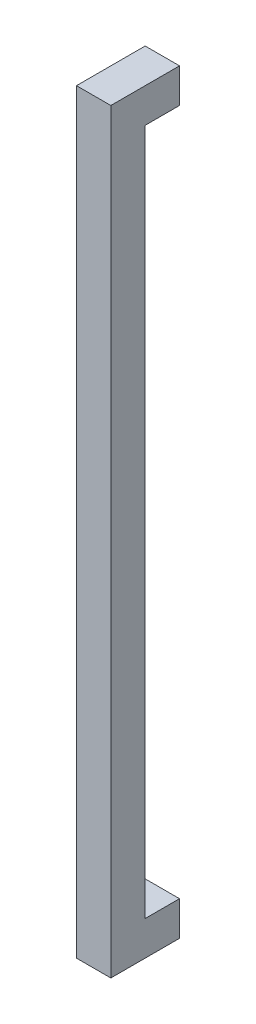
# Autodesk Inventor part: ReinforcerLarge
Saved by Autodesk Inventor 2027 (Build 310192000, 192)
## iProperties
Created: 2026-04-15
Part Number: ReinforcerLarge
Material: Generic
Document SubType Name: Modeling
Designer: Tueha
Density: 1 g/cm^3
Appearance: Default
Author: Tueha
Autodesk Inventor part; units mm, degrees
ref_plane "YZ Plane" through (0, 0, 0) normal (1, 0, 0) x (0, 1, 0)
ref_plane "XZ Plane" through (0, 0, 0) normal (0, 1, 0) x (-1, 0, 0)
ref_plane "XY Plane" through (0, 0, 0) normal (0, 0, 1) x (1, 0, 0)
sketch "Sketch1" plane through (0, 0, 0) normal (0, 0, 1) x (1, 0, 0)
  line L0 (538.5222, 35.1205) -> (532.3222, 35.1205) projected
  line L1 (538.5222, 52.0205) -> (538.5222, 35.1205) projected
  line L2 (538.5222, 52.0205) -> (246.9222, 52.0205) projected
  line L3 (246.9222, 52.0205) -> (246.9222, 58.0205) projected
  line L4 (246.9222, 58.0205) -> (538.5222, 58.0205) projected
  line L5 (538.5222, 74.9205) -> (538.5222, 58.0205) projected
  line L6 (523.1184, 74.9205) -> (538.5222, 74.9205) projected
  line L7 (517.9222, 77.9205) -> (523.1184, 74.9205) projected
  line L8 (517.9222, 74.9205) -> (517.9222, 77.9205) projected
  arc A0 (515.9222, 74.9205) -> (517.9222, 74.9205) centre (516.9222, 74.9205) ccw projected
  line L9 (515.9222, 77.9205) -> (515.9222, 74.9205) projected
  line L10 (510.7261, 74.9205) -> (515.9222, 77.9205) projected
  line L11 (494.3184, 74.9205) -> (510.7261, 74.9205) projected
  line L12 (489.1222, 77.9205) -> (494.3184, 74.9205) projected
  line L13 (489.1222, 74.9205) -> (489.1222, 77.9205) projected
  arc A1 (487.1222, 74.9205) -> (489.1222, 74.9205) centre (488.1222, 74.9205) ccw projected
  line L14 (487.1222, 77.9205) -> (487.1222, 74.9205) projected
  line L15 (481.9261, 74.9205) -> (487.1222, 77.9205) projected
  line L16 (465.5184, 74.9205) -> (481.9261, 74.9205) projected
  line L17 (460.3222, 77.9205) -> (465.5184, 74.9205) projected
  line L18 (460.3222, 74.9205) -> (460.3222, 77.9205) projected
  arc A2 (458.3222, 74.9205) -> (460.3222, 74.9205) centre (459.3222, 74.9205) ccw projected
  line L19 (458.3222, 77.9205) -> (458.3222, 74.9205) projected
  line L20 (453.1261, 74.9205) -> (458.3222, 77.9205) projected
  line L21 (436.7184, 74.9205) -> (453.1261, 74.9205) projected
  line L22 (431.5222, 77.9205) -> (436.7184, 74.9205) projected
  line L23 (431.5222, 74.9205) -> (431.5222, 77.9205) projected
  arc A3 (429.5222, 74.9205) -> (431.5222, 74.9205) centre (430.5222, 74.9205) ccw projected
  line L24 (429.5222, 77.9205) -> (429.5222, 74.9205) projected
  line L25 (424.3261, 74.9205) -> (429.5222, 77.9205) projected
  line L26 (407.9184, 74.9205) -> (424.3261, 74.9205) projected
  line L27 (402.7222, 77.9205) -> (407.9184, 74.9205) projected
  line L28 (402.7222, 74.9205) -> (402.7222, 77.9205) projected
  arc A4 (400.7222, 74.9205) -> (402.7222, 74.9205) centre (401.7222, 74.9205) ccw projected
  line L29 (400.7222, 77.9205) -> (400.7222, 74.9205) projected
  line L30 (395.5261, 74.9205) -> (400.7222, 77.9205) projected
  line L31 (379.1184, 74.9205) -> (395.5261, 74.9205) projected
  line L32 (373.9222, 77.9205) -> (379.1184, 74.9205) projected
  line L33 (373.9222, 74.9205) -> (373.9222, 77.9205) projected
  arc A5 (371.9222, 74.9205) -> (373.9222, 74.9205) centre (372.9222, 74.9205) ccw projected
  line L34 (371.9222, 77.9205) -> (371.9222, 74.9205) projected
  line L35 (366.7261, 74.9205) -> (371.9222, 77.9205) projected
  line L36 (350.3184, 74.9205) -> (366.7261, 74.9205) projected
  line L37 (345.1222, 77.9205) -> (350.3184, 74.9205) projected
  line L38 (345.1222, 74.9205) -> (345.1222, 77.9205) projected
  arc A6 (343.1222, 74.9205) -> (345.1222, 74.9205) centre (344.1222, 74.9205) ccw projected
  line L39 (343.1222, 77.9205) -> (343.1222, 74.9205) projected
  line L40 (337.9261, 74.9205) -> (343.1222, 77.9205) projected
  line L41 (321.5184, 74.9205) -> (337.9261, 74.9205) projected
  line L42 (316.3222, 77.9205) -> (321.5184, 74.9205) projected
  line L43 (316.3222, 74.9205) -> (316.3222, 77.9205) projected
  arc A7 (314.3222, 74.9205) -> (316.3222, 74.9205) centre (315.3222, 74.9205) ccw projected
  line L44 (314.3222, 77.9205) -> (314.3222, 74.9205) projected
  line L45 (309.1261, 74.9205) -> (314.3222, 77.9205) projected
  line L46 (292.7184, 74.9205) -> (309.1261, 74.9205) projected
  line L47 (287.5222, 77.9205) -> (292.7184, 74.9205) projected
  line L48 (287.5222, 74.9205) -> (287.5222, 77.9205) projected
  arc A8 (285.5222, 74.9205) -> (287.5222, 74.9205) centre (286.5222, 74.9205) ccw projected
  line L49 (285.5222, 77.9205) -> (285.5222, 74.9205) projected
  line L50 (280.3261, 74.9205) -> (285.5222, 77.9205) projected
  line L51 (263.9184, 74.9205) -> (280.3261, 74.9205) projected
  line L52 (258.7222, 77.9205) -> (263.9184, 74.9205) projected
  line L53 (258.7222, 74.9205) -> (258.7222, 77.9205) projected
  arc A9 (256.7222, 74.9205) -> (258.7222, 74.9205) centre (257.7222, 74.9205) ccw projected
  line L54 (256.7222, 77.9205) -> (256.7222, 74.9205) projected
  line L55 (251.5261, 74.9205) -> (256.7222, 77.9205) projected
  line L56 (235.1184, 74.9205) -> (251.5261, 74.9205) projected
  line L57 (229.9222, 77.9205) -> (235.1184, 74.9205) projected
  line L58 (229.9222, 74.9205) -> (229.9222, 77.9205) projected
  arc A10 (227.9222, 74.9205) -> (229.9222, 74.9205) centre (228.9222, 74.9205) ccw projected
  line L59 (227.9222, 77.9205) -> (227.9222, 74.9205) projected
  line L60 (222.7261, 74.9205) -> (227.9222, 77.9205) projected
  line L61 (206.3184, 74.9205) -> (222.7261, 74.9205) projected
  line L62 (201.1222, 77.9205) -> (206.3184, 74.9205) projected
  line L63 (201.1222, 74.9205) -> (201.1222, 77.9205) projected
  arc A11 (199.1222, 74.9205) -> (201.1222, 74.9205) centre (200.1222, 74.9205) ccw projected
  line L64 (199.1222, 77.9205) -> (199.1222, 74.9205) projected
  line L65 (193.9261, 74.9205) -> (199.1222, 77.9205) projected
  line L66 (177.5184, 74.9205) -> (193.9261, 74.9205) projected
  line L67 (172.3222, 77.9205) -> (177.5184, 74.9205) projected
  line L68 (172.3222, 74.9205) -> (172.3222, 77.9205) projected
  arc A12 (170.3222, 74.9205) -> (172.3222, 74.9205) centre (171.3222, 74.9205) ccw projected
  line L69 (170.3222, 77.9205) -> (170.3222, 74.9205) projected
  line L70 (165.1261, 74.9205) -> (170.3222, 77.9205) projected
  line L71 (148.7184, 74.9205) -> (165.1261, 74.9205) projected
  line L72 (143.5222, 77.9205) -> (148.7184, 74.9205) projected
  line L73 (143.5222, 74.9205) -> (143.5222, 77.9205) projected
  arc A13 (141.5222, 74.9205) -> (143.5222, 74.9205) centre (142.5222, 74.9205) ccw projected
  line L74 (141.5222, 77.9205) -> (141.5222, 74.9205) projected
  line L75 (136.3261, 74.9205) -> (141.5222, 77.9205) projected
  line L76 (119.9184, 74.9205) -> (136.3261, 74.9205) projected
  line L77 (114.7222, 77.9205) -> (119.9184, 74.9205) projected
  line L78 (114.7222, 74.9205) -> (114.7222, 77.9205) projected
  arc A14 (112.7222, 74.9205) -> (114.7222, 74.9205) centre (113.7222, 74.9205) ccw projected
  line L79 (112.7222, 77.9205) -> (112.7222, 74.9205) projected
  line L80 (107.5261, 74.9205) -> (112.7222, 77.9205) projected
  line L81 (91.1184, 74.9205) -> (107.5261, 74.9205) projected
  line L82 (85.9222, 77.9205) -> (91.1184, 74.9205) projected
  line L83 (85.9222, 74.9205) -> (85.9222, 77.9205) projected
  arc A15 (83.9222, 74.9205) -> (85.9222, 74.9205) centre (84.9222, 74.9205) ccw projected
  line L84 (83.9222, 77.9205) -> (83.9222, 74.9205) projected
  line L85 (78.7261, 74.9205) -> (83.9222, 77.9205) projected
  line L86 (62.3184, 74.9205) -> (78.7261, 74.9205) projected
  line L87 (57.1222, 77.9205) -> (62.3184, 74.9205) projected
  line L88 (57.1222, 74.9205) -> (57.1222, 77.9205) projected
  arc A16 (55.1222, 74.9205) -> (57.1222, 74.9205) centre (56.1222, 74.9205) ccw projected
  line L89 (55.1222, 77.9205) -> (55.1222, 74.9205) projected
  line L90 (49.9261, 74.9205) -> (55.1222, 77.9205) projected
  line L91 (33.5184, 74.9205) -> (49.9261, 74.9205) projected
  line L92 (28.3222, 77.9205) -> (33.5184, 74.9205) projected
  line L93 (28.3222, 74.9205) -> (28.3222, 77.9205) projected
  arc A17 (26.3222, 74.9205) -> (28.3222, 74.9205) centre (27.3222, 74.9205) ccw projected
  line L94 (26.3222, 77.9205) -> (26.3222, 74.9205) projected
  line L95 (21.1261, 74.9205) -> (26.3222, 77.9205) projected
  line L96 (4.7184, 74.9205) -> (21.1261, 74.9205) projected
  line L97 (-0.4778, 77.9205) -> (4.7184, 74.9205) projected
  line L98 (-0.4778, 74.9205) -> (-0.4778, 77.9205) projected
  arc A18 (-2.4778, 74.9205) -> (-0.4778, 74.9205) centre (-1.4778, 74.9205) ccw projected
  line L99 (-2.4778, 77.9205) -> (-2.4778, 74.9205) projected
  line L100 (-7.6739, 74.9205) -> (-2.4778, 77.9205) projected
  line L101 (-24.0816, 74.9205) -> (-7.6739, 74.9205) projected
  line L102 (-29.2778, 77.9205) -> (-24.0816, 74.9205) projected
  line L103 (-29.2778, 74.9205) -> (-29.2778, 77.9205) projected
  arc A19 (-31.2778, 74.9205) -> (-29.2778, 74.9205) centre (-30.2778, 74.9205) ccw projected
  line L104 (-31.2778, 77.9205) -> (-31.2778, 74.9205) projected
  line L105 (-36.4739, 74.9205) -> (-31.2778, 77.9205) projected
  line L106 (-36.4739, 74.9205) -> (-44.6778, 74.9205) projected
  line L107 (-44.6778, 35.1205) -> (-44.6778, 74.9205) projected
  line L108 (-22.0739, 35.1205) -> (-44.6778, 35.1205) projected
  line L109 (-16.8778, 32.1205) -> (-22.0739, 35.1205) projected
  line L110 (-16.8778, 35.1205) -> (-16.8778, 32.1205) projected
  arc A20 (-14.8778, 35.1205) -> (-16.8778, 35.1205) centre (-15.8778, 35.1205) ccw projected
  line L111 (-14.8778, 32.1205) -> (-14.8778, 35.1205) projected
  line L112 (-9.6816, 35.1205) -> (-14.8778, 32.1205) projected
  line L113 (6.7261, 35.1205) -> (-9.6816, 35.1205) projected
  line L114 (11.9222, 32.1205) -> (6.7261, 35.1205) projected
  line L115 (11.9222, 35.1205) -> (11.9222, 32.1205) projected
  arc A21 (13.9222, 35.1205) -> (11.9222, 35.1205) centre (12.9222, 35.1205) ccw projected
  line L116 (13.9222, 32.1205) -> (13.9222, 35.1205) projected
  line L117 (19.1184, 35.1205) -> (13.9222, 32.1205) projected
  line L118 (35.5261, 35.1205) -> (19.1184, 35.1205) projected
  line L119 (40.7222, 32.1205) -> (35.5261, 35.1205) projected
  line L120 (40.7222, 35.1205) -> (40.7222, 32.1205) projected
  arc A22 (42.7222, 35.1205) -> (40.7222, 35.1205) centre (41.7222, 35.1205) ccw projected
  line L121 (42.7222, 32.1205) -> (42.7222, 35.1205) projected
  line L122 (47.9184, 35.1205) -> (42.7222, 32.1205) projected
  line L123 (64.3261, 35.1205) -> (47.9184, 35.1205) projected
  line L124 (69.5222, 32.1205) -> (64.3261, 35.1205) projected
  line L125 (69.5222, 35.1205) -> (69.5222, 32.1205) projected
  arc A23 (71.5222, 35.1205) -> (69.5222, 35.1205) centre (70.5222, 35.1205) ccw projected
  line L126 (71.5222, 32.1205) -> (71.5222, 35.1205) projected
  line L127 (76.7184, 35.1205) -> (71.5222, 32.1205) projected
  line L128 (93.1261, 35.1205) -> (76.7184, 35.1205) projected
  line L129 (98.3222, 32.1205) -> (93.1261, 35.1205) projected
  line L130 (98.3222, 35.1205) -> (98.3222, 32.1205) projected
  arc A24 (100.3222, 35.1205) -> (98.3222, 35.1205) centre (99.3222, 35.1205) ccw projected
  line L131 (100.3222, 32.1205) -> (100.3222, 35.1205) projected
  line L132 (105.5184, 35.1205) -> (100.3222, 32.1205) projected
  line L133 (121.9261, 35.1205) -> (105.5184, 35.1205) projected
  line L134 (127.1222, 32.1205) -> (121.9261, 35.1205) projected
  line L135 (127.1222, 35.1205) -> (127.1222, 32.1205) projected
  arc A25 (129.1222, 35.1205) -> (127.1222, 35.1205) centre (128.1222, 35.1205) ccw projected
  line L136 (129.1222, 32.1205) -> (129.1222, 35.1205) projected
  line L137 (134.3184, 35.1205) -> (129.1222, 32.1205) projected
  line L138 (150.7261, 35.1205) -> (134.3184, 35.1205) projected
  line L139 (155.9222, 32.1205) -> (150.7261, 35.1205) projected
  line L140 (155.9222, 35.1205) -> (155.9222, 32.1205) projected
  arc A26 (157.9222, 35.1205) -> (155.9222, 35.1205) centre (156.9222, 35.1205) ccw projected
  line L141 (157.9222, 32.1205) -> (157.9222, 35.1205) projected
  line L142 (163.1184, 35.1205) -> (157.9222, 32.1205) projected
  line L143 (179.5261, 35.1205) -> (163.1184, 35.1205) projected
  line L144 (184.7222, 32.1205) -> (179.5261, 35.1205) projected
  line L145 (184.7222, 35.1205) -> (184.7222, 32.1205) projected
  arc A27 (186.7222, 35.1205) -> (184.7222, 35.1205) centre (185.7222, 35.1205) ccw projected
  line L146 (186.7222, 32.1205) -> (186.7222, 35.1205) projected
  line L147 (191.9184, 35.1205) -> (186.7222, 32.1205) projected
  line L148 (208.3261, 35.1205) -> (191.9184, 35.1205) projected
  line L149 (213.5222, 32.1205) -> (208.3261, 35.1205) projected
  line L150 (213.5222, 35.1205) -> (213.5222, 32.1205) projected
  arc A28 (215.5222, 35.1205) -> (213.5222, 35.1205) centre (214.5222, 35.1205) ccw projected
  line L151 (215.5222, 32.1205) -> (215.5222, 35.1205) projected
  line L152 (220.7184, 35.1205) -> (215.5222, 32.1205) projected
  line L153 (237.1261, 35.1205) -> (220.7184, 35.1205) projected
  line L154 (242.3222, 32.1205) -> (237.1261, 35.1205) projected
  line L155 (242.3222, 35.1205) -> (242.3222, 32.1205) projected
  arc A29 (244.3222, 35.1205) -> (242.3222, 35.1205) centre (243.3222, 35.1205) ccw projected
  line L156 (244.3222, 32.1205) -> (244.3222, 35.1205) projected
  line L157 (249.5184, 35.1205) -> (244.3222, 32.1205) projected
  line L158 (265.9261, 35.1205) -> (249.5184, 35.1205) projected
  line L159 (271.1222, 32.1205) -> (265.9261, 35.1205) projected
  line L160 (271.1222, 35.1205) -> (271.1222, 32.1205) projected
  arc A30 (273.1222, 35.1205) -> (271.1222, 35.1205) centre (272.1222, 35.1205) ccw projected
  line L161 (273.1222, 32.1205) -> (273.1222, 35.1205) projected
  line L162 (278.3184, 35.1205) -> (273.1222, 32.1205) projected
  line L163 (294.7261, 35.1205) -> (278.3184, 35.1205) projected
  line L164 (299.9222, 32.1205) -> (294.7261, 35.1205) projected
  line L165 (299.9222, 35.1205) -> (299.9222, 32.1205) projected
  arc A31 (301.9222, 35.1205) -> (299.9222, 35.1205) centre (300.9222, 35.1205) ccw projected
  line L166 (301.9222, 32.1205) -> (301.9222, 35.1205) projected
  line L167 (307.1184, 35.1205) -> (301.9222, 32.1205) projected
  line L168 (323.5261, 35.1205) -> (307.1184, 35.1205) projected
  line L169 (328.7222, 32.1205) -> (323.5261, 35.1205) projected
  line L170 (328.7222, 35.1205) -> (328.7222, 32.1205) projected
  arc A32 (330.7222, 35.1205) -> (328.7222, 35.1205) centre (329.7222, 35.1205) ccw projected
  line L171 (330.7222, 32.1205) -> (330.7222, 35.1205) projected
  line L172 (335.9184, 35.1205) -> (330.7222, 32.1205) projected
  line L173 (352.3261, 35.1205) -> (335.9184, 35.1205) projected
  line L174 (357.5222, 32.1205) -> (352.3261, 35.1205) projected
  line L175 (357.5222, 35.1205) -> (357.5222, 32.1205) projected
  arc A33 (359.5222, 35.1205) -> (357.5222, 35.1205) centre (358.5222, 35.1205) ccw projected
  line L176 (359.5222, 32.1205) -> (359.5222, 35.1205) projected
  line L177 (364.7184, 35.1205) -> (359.5222, 32.1205) projected
  line L178 (381.1261, 35.1205) -> (364.7184, 35.1205) projected
  line L179 (386.3222, 32.1205) -> (381.1261, 35.1205) projected
  line L180 (386.3222, 35.1205) -> (386.3222, 32.1205) projected
  arc A34 (388.3222, 35.1205) -> (386.3222, 35.1205) centre (387.3222, 35.1205) ccw projected
  line L181 (388.3222, 32.1205) -> (388.3222, 35.1205) projected
  line L182 (393.5184, 35.1205) -> (388.3222, 32.1205) projected
  line L183 (409.9261, 35.1205) -> (393.5184, 35.1205) projected
  line L184 (415.1222, 32.1205) -> (409.9261, 35.1205) projected
  line L185 (415.1222, 35.1205) -> (415.1222, 32.1205) projected
  arc A35 (417.1222, 35.1205) -> (415.1222, 35.1205) centre (416.1222, 35.1205) ccw projected
  line L186 (417.1222, 32.1205) -> (417.1222, 35.1205) projected
  line L187 (422.3184, 35.1205) -> (417.1222, 32.1205) projected
  line L188 (438.7261, 35.1205) -> (422.3184, 35.1205) projected
  line L189 (443.9222, 32.1205) -> (438.7261, 35.1205) projected
  line L190 (443.9222, 35.1205) -> (443.9222, 32.1205) projected
  arc A36 (445.9222, 35.1205) -> (443.9222, 35.1205) centre (444.9222, 35.1205) ccw projected
  line L191 (445.9222, 32.1205) -> (445.9222, 35.1205) projected
  line L192 (451.1184, 35.1205) -> (445.9222, 32.1205) projected
  line L193 (467.5261, 35.1205) -> (451.1184, 35.1205) projected
  line L194 (472.7222, 32.1205) -> (467.5261, 35.1205) projected
  line L195 (472.7222, 35.1205) -> (472.7222, 32.1205) projected
  arc A37 (474.7222, 35.1205) -> (472.7222, 35.1205) centre (473.7222, 35.1205) ccw projected
  line L196 (474.7222, 32.1205) -> (474.7222, 35.1205) projected
  line L197 (479.9184, 35.1205) -> (474.7222, 32.1205) projected
  line L198 (496.3261, 35.1205) -> (479.9184, 35.1205) projected
  line L199 (501.5222, 32.1205) -> (496.3261, 35.1205) projected
  line L200 (501.5222, 35.1205) -> (501.5222, 32.1205) projected
  arc A38 (503.5222, 35.1205) -> (501.5222, 35.1205) centre (502.5222, 35.1205) ccw projected
  line L201 (503.5222, 32.1205) -> (503.5222, 35.1205) projected
  line L202 (508.7184, 35.1205) -> (503.5222, 32.1205) projected
  line L203 (525.1261, 35.1205) -> (508.7184, 35.1205) projected
  line L204 (530.3222, 32.1205) -> (525.1261, 35.1205) projected
  line L205 (530.3222, 35.1205) -> (530.3222, 32.1205) projected
  arc A39 (532.3222, 35.1205) -> (530.3222, 35.1205) centre (531.3222, 35.1205) ccw projected
  line L206 (-15.2778, 46.0205) -> (-9.2778, 46.0205) projected
  line L207 (-9.2778, 46.0205) -> (-9.2778, 40.0205) projected
  line L208 (-9.2778, 40.0205) -> (-15.2778, 40.0205) projected
  line L209 (-15.2778, 40.0205) -> (-15.2778, 46.0205) projected
  line L210 (-15.2778, 64.0205) -> (-15.2778, 70.0205) projected
  line L211 (-15.2778, 70.0205) -> (-9.2778, 70.0205) projected
  line L212 (-9.2778, 70.0205) -> (-9.2778, 64.0205) projected
  line L213 (-9.2778, 64.0205) -> (-15.2778, 64.0205) projected
  line L214 (42.3222, 46.0205) -> (48.3222, 46.0205) projected
  line L215 (48.3222, 46.0205) -> (48.3222, 40.0205) projected
  line L216 (48.3222, 40.0205) -> (42.3222, 40.0205) projected
  line L217 (42.3222, 40.0205) -> (42.3222, 46.0205) projected
  line L218 (42.3222, 64.0205) -> (42.3222, 70.0205) projected
  line L219 (42.3222, 70.0205) -> (48.3222, 70.0205) projected
  line L220 (48.3222, 70.0205) -> (48.3222, 64.0205) projected
  line L221 (48.3222, 64.0205) -> (42.3222, 64.0205) projected
  line L222 (99.9222, 46.0205) -> (105.9222, 46.0205) projected
  line L223 (105.9222, 46.0205) -> (105.9222, 40.0205) projected
  line L224 (105.9222, 40.0205) -> (99.9222, 40.0205) projected
  line L225 (99.9222, 40.0205) -> (99.9222, 46.0205) projected
  line L226 (99.9222, 64.0205) -> (99.9222, 70.0205) projected
  line L227 (99.9222, 70.0205) -> (105.9222, 70.0205) projected
  line L228 (105.9222, 70.0205) -> (105.9222, 64.0205) projected
  line L229 (105.9222, 64.0205) -> (99.9222, 64.0205) projected
  line L230 (157.5222, 46.0205) -> (163.5222, 46.0205) projected
  line L231 (163.5222, 46.0205) -> (163.5222, 40.0205) projected
  line L232 (163.5222, 40.0205) -> (157.5222, 40.0205) projected
  line L233 (157.5222, 40.0205) -> (157.5222, 46.0205) projected
  line L234 (157.5222, 64.0205) -> (157.5222, 70.0205) projected
  line L235 (157.5222, 70.0205) -> (163.5222, 70.0205) projected
  line L236 (163.5222, 70.0205) -> (163.5222, 64.0205) projected
  line L237 (163.5222, 64.0205) -> (157.5222, 64.0205) projected
  line L238 (215.1222, 46.0205) -> (221.1222, 46.0205) projected
  line L239 (221.1222, 46.0205) -> (221.1222, 40.0205) projected
  line L240 (221.1222, 40.0205) -> (215.1222, 40.0205) projected
  line L241 (215.1222, 40.0205) -> (215.1222, 46.0205) projected
  line L242 (215.1222, 64.0205) -> (215.1222, 70.0205) projected
  line L243 (215.1222, 70.0205) -> (221.1222, 70.0205) projected
  line L244 (221.1222, 70.0205) -> (221.1222, 64.0205) projected
  line L245 (221.1222, 64.0205) -> (215.1222, 64.0205) projected
  line L246 (272.7222, 46.0205) -> (278.7222, 46.0205) projected
  line L247 (278.7222, 46.0205) -> (278.7222, 40.0205) projected
  line L248 (278.7222, 40.0205) -> (272.7222, 40.0205) projected
  line L249 (272.7222, 40.0205) -> (272.7222, 46.0205) projected
  line L250 (272.7222, 64.0205) -> (272.7222, 70.0205) projected
  line L251 (272.7222, 70.0205) -> (278.7222, 70.0205) projected
  line L252 (278.7222, 70.0205) -> (278.7222, 64.0205) projected
  line L253 (278.7222, 64.0205) -> (272.7222, 64.0205) projected
  line L254 (330.3222, 46.0205) -> (336.3222, 46.0205) projected
  line L255 (336.3222, 46.0205) -> (336.3222, 40.0205) projected
  line L256 (336.3222, 40.0205) -> (330.3222, 40.0205) projected
  line L257 (330.3222, 40.0205) -> (330.3222, 46.0205) projected
  line L258 (330.3222, 64.0205) -> (330.3222, 70.0205) projected
  line L259 (330.3222, 70.0205) -> (336.3222, 70.0205) projected
  line L260 (336.3222, 70.0205) -> (336.3222, 64.0205) projected
  line L261 (336.3222, 64.0205) -> (330.3222, 64.0205) projected
  line L262 (387.9222, 46.0205) -> (393.9222, 46.0205) projected
  line L263 (393.9222, 46.0205) -> (393.9222, 40.0205) projected
  line L264 (393.9222, 40.0205) -> (387.9222, 40.0205) projected
  line L265 (387.9222, 40.0205) -> (387.9222, 46.0205) projected
  line L266 (387.9222, 64.0205) -> (387.9222, 70.0205) projected
  line L267 (387.9222, 70.0205) -> (393.9222, 70.0205) projected
  line L268 (393.9222, 70.0205) -> (393.9222, 64.0205) projected
  line L269 (393.9222, 64.0205) -> (387.9222, 64.0205) projected
  line L270 (445.5222, 46.0205) -> (451.5222, 46.0205) projected
  line L271 (451.5222, 46.0205) -> (451.5222, 40.0205) projected
  line L272 (451.5222, 40.0205) -> (445.5222, 40.0205) projected
  line L273 (445.5222, 40.0205) -> (445.5222, 46.0205) projected
  line L274 (445.5222, 64.0205) -> (445.5222, 70.0205) projected
  line L275 (445.5222, 70.0205) -> (451.5222, 70.0205) projected
  line L276 (451.5222, 70.0205) -> (451.5222, 64.0205) projected
  line L277 (451.5222, 64.0205) -> (445.5222, 64.0205) projected
  line L278 (503.1222, 46.0205) -> (509.1222, 46.0205) projected
  line L279 (509.1222, 46.0205) -> (509.1222, 40.0205) projected
  line L280 (509.1222, 40.0205) -> (503.1222, 40.0205) projected
  line L281 (503.1222, 40.0205) -> (503.1222, 46.0205) projected
  line L282 (503.1222, 64.0205) -> (503.1222, 70.0205) projected
  line L283 (503.1222, 70.0205) -> (509.1222, 70.0205) projected
  line L284 (509.1222, 70.0205) -> (509.1222, 64.0205) projected
  line L285 (509.1222, 64.0205) -> (503.1222, 64.0205) projected
  line L286 (538.5222, -114.8795) -> (532.3222, -114.8795) projected
  line L287 (538.5222, -97.9795) -> (538.5222, -114.8795) projected
  line L288 (538.5222, -97.9795) -> (246.9222, -97.9795) projected
  line L289 (246.9222, -97.9795) -> (246.9222, -91.9795) projected
  line L290 (246.9222, -91.9795) -> (538.5222, -91.9795) projected
  line L291 (538.5222, -75.0795) -> (538.5222, -91.9795) projected
  line L292 (523.1184, -75.0795) -> (538.5222, -75.0795) projected
  line L293 (517.9222, -72.0795) -> (523.1184, -75.0795) projected
  line L294 (517.9222, -75.0795) -> (517.9222, -72.0795) projected
  arc A40 (515.9222, -75.0795) -> (517.9222, -75.0795) centre (516.9222, -75.0795) ccw projected
  line L295 (515.9222, -72.0795) -> (515.9222, -75.0795) projected
  line L296 (510.7261, -75.0795) -> (515.9222, -72.0795) projected
  line L297 (494.3184, -75.0795) -> (510.7261, -75.0795) projected
  line L298 (489.1222, -72.0795) -> (494.3184, -75.0795) projected
  line L299 (489.1222, -75.0795) -> (489.1222, -72.0795) projected
  arc A41 (487.1222, -75.0795) -> (489.1222, -75.0795) centre (488.1222, -75.0795) ccw projected
  line L300 (487.1222, -72.0795) -> (487.1222, -75.0795) projected
  line L301 (481.9261, -75.0795) -> (487.1222, -72.0795) projected
  line L302 (465.5184, -75.0795) -> (481.9261, -75.0795) projected
  line L303 (460.3222, -72.0795) -> (465.5184, -75.0795) projected
  line L304 (460.3222, -75.0795) -> (460.3222, -72.0795) projected
  arc A42 (458.3222, -75.0795) -> (460.3222, -75.0795) centre (459.3222, -75.0795) ccw projected
  line L305 (458.3222, -72.0795) -> (458.3222, -75.0795) projected
  line L306 (453.1261, -75.0795) -> (458.3222, -72.0795) projected
  line L307 (436.7184, -75.0795) -> (453.1261, -75.0795) projected
  line L308 (431.5222, -72.0795) -> (436.7184, -75.0795) projected
  line L309 (431.5222, -75.0795) -> (431.5222, -72.0795) projected
  arc A43 (429.5222, -75.0795) -> (431.5222, -75.0795) centre (430.5222, -75.0795) ccw projected
  line L310 (429.5222, -72.0795) -> (429.5222, -75.0795) projected
  line L311 (424.3261, -75.0795) -> (429.5222, -72.0795) projected
  line L312 (407.9184, -75.0795) -> (424.3261, -75.0795) projected
  line L313 (402.7222, -72.0795) -> (407.9184, -75.0795) projected
  line L314 (402.7222, -75.0795) -> (402.7222, -72.0795) projected
  arc A44 (400.7222, -75.0795) -> (402.7222, -75.0795) centre (401.7222, -75.0795) ccw projected
  line L315 (400.7222, -72.0795) -> (400.7222, -75.0795) projected
  line L316 (395.5261, -75.0795) -> (400.7222, -72.0795) projected
  line L317 (379.1184, -75.0795) -> (395.5261, -75.0795) projected
  line L318 (373.9222, -72.0795) -> (379.1184, -75.0795) projected
  line L319 (373.9222, -75.0795) -> (373.9222, -72.0795) projected
  arc A45 (371.9222, -75.0795) -> (373.9222, -75.0795) centre (372.9222, -75.0795) ccw projected
  line L320 (371.9222, -72.0795) -> (371.9222, -75.0795) projected
  line L321 (366.7261, -75.0795) -> (371.9222, -72.0795) projected
  line L322 (350.3184, -75.0795) -> (366.7261, -75.0795) projected
  line L323 (345.1222, -72.0795) -> (350.3184, -75.0795) projected
  line L324 (345.1222, -75.0795) -> (345.1222, -72.0795) projected
  arc A46 (343.1222, -75.0795) -> (345.1222, -75.0795) centre (344.1222, -75.0795) ccw projected
  line L325 (343.1222, -72.0795) -> (343.1222, -75.0795) projected
  line L326 (337.9261, -75.0795) -> (343.1222, -72.0795) projected
  line L327 (321.5184, -75.0795) -> (337.9261, -75.0795) projected
  line L328 (316.3222, -72.0795) -> (321.5184, -75.0795) projected
  line L329 (316.3222, -75.0795) -> (316.3222, -72.0795) projected
  arc A47 (314.3222, -75.0795) -> (316.3222, -75.0795) centre (315.3222, -75.0795) ccw projected
  line L330 (314.3222, -72.0795) -> (314.3222, -75.0795) projected
  line L331 (309.1261, -75.0795) -> (314.3222, -72.0795) projected
  line L332 (292.7184, -75.0795) -> (309.1261, -75.0795) projected
  line L333 (287.5222, -72.0795) -> (292.7184, -75.0795) projected
  line L334 (287.5222, -75.0795) -> (287.5222, -72.0795) projected
  arc A48 (285.5222, -75.0795) -> (287.5222, -75.0795) centre (286.5222, -75.0795) ccw projected
  line L335 (285.5222, -72.0795) -> (285.5222, -75.0795) projected
  line L336 (280.3261, -75.0795) -> (285.5222, -72.0795) projected
  line L337 (263.9184, -75.0795) -> (280.3261, -75.0795) projected
  line L338 (258.7222, -72.0795) -> (263.9184, -75.0795) projected
  line L339 (258.7222, -75.0795) -> (258.7222, -72.0795) projected
  arc A49 (256.7222, -75.0795) -> (258.7222, -75.0795) centre (257.7222, -75.0795) ccw projected
  line L340 (256.7222, -72.0795) -> (256.7222, -75.0795) projected
  line L341 (251.5261, -75.0795) -> (256.7222, -72.0795) projected
  line L342 (235.1184, -75.0795) -> (251.5261, -75.0795) projected
  line L343 (229.9222, -72.0795) -> (235.1184, -75.0795) projected
  line L344 (229.9222, -75.0795) -> (229.9222, -72.0795) projected
  arc A50 (227.9222, -75.0795) -> (229.9222, -75.0795) centre (228.9222, -75.0795) ccw projected
  line L345 (227.9222, -72.0795) -> (227.9222, -75.0795) projected
  line L346 (222.7261, -75.0795) -> (227.9222, -72.0795) projected
  line L347 (206.3184, -75.0795) -> (222.7261, -75.0795) projected
  line L348 (201.1222, -72.0795) -> (206.3184, -75.0795) projected
  line L349 (201.1222, -75.0795) -> (201.1222, -72.0795) projected
  arc A51 (199.1222, -75.0795) -> (201.1222, -75.0795) centre (200.1222, -75.0795) ccw projected
  line L350 (199.1222, -72.0795) -> (199.1222, -75.0795) projected
  line L351 (193.9261, -75.0795) -> (199.1222, -72.0795) projected
  line L352 (177.5184, -75.0795) -> (193.9261, -75.0795) projected
  line L353 (172.3222, -72.0795) -> (177.5184, -75.0795) projected
  line L354 (172.3222, -75.0795) -> (172.3222, -72.0795) projected
  arc A52 (170.3222, -75.0795) -> (172.3222, -75.0795) centre (171.3222, -75.0795) ccw projected
  line L355 (170.3222, -72.0795) -> (170.3222, -75.0795) projected
  line L356 (165.1261, -75.0795) -> (170.3222, -72.0795) projected
  line L357 (148.7184, -75.0795) -> (165.1261, -75.0795) projected
  line L358 (143.5222, -72.0795) -> (148.7184, -75.0795) projected
  line L359 (143.5222, -75.0795) -> (143.5222, -72.0795) projected
  arc A53 (141.5222, -75.0795) -> (143.5222, -75.0795) centre (142.5222, -75.0795) ccw projected
  line L360 (141.5222, -72.0795) -> (141.5222, -75.0795) projected
  line L361 (136.3261, -75.0795) -> (141.5222, -72.0795) projected
  line L362 (119.9184, -75.0795) -> (136.3261, -75.0795) projected
  line L363 (114.7222, -72.0795) -> (119.9184, -75.0795) projected
  line L364 (114.7222, -75.0795) -> (114.7222, -72.0795) projected
  arc A54 (112.7222, -75.0795) -> (114.7222, -75.0795) centre (113.7222, -75.0795) ccw projected
  line L365 (112.7222, -72.0795) -> (112.7222, -75.0795) projected
  line L366 (107.5261, -75.0795) -> (112.7222, -72.0795) projected
  line L367 (91.1184, -75.0795) -> (107.5261, -75.0795) projected
  line L368 (85.9222, -72.0795) -> (91.1184, -75.0795) projected
  line L369 (85.9222, -75.0795) -> (85.9222, -72.0795) projected
  arc A55 (83.9222, -75.0795) -> (85.9222, -75.0795) centre (84.9222, -75.0795) ccw projected
  line L370 (83.9222, -72.0795) -> (83.9222, -75.0795) projected
  line L371 (78.7261, -75.0795) -> (83.9222, -72.0795) projected
  line L372 (62.3184, -75.0795) -> (78.7261, -75.0795) projected
  line L373 (57.1222, -72.0795) -> (62.3184, -75.0795) projected
  line L374 (57.1222, -75.0795) -> (57.1222, -72.0795) projected
  arc A56 (55.1222, -75.0795) -> (57.1222, -75.0795) centre (56.1222, -75.0795) ccw projected
  line L375 (55.1222, -72.0795) -> (55.1222, -75.0795) projected
  line L376 (49.9261, -75.0795) -> (55.1222, -72.0795) projected
  line L377 (33.5184, -75.0795) -> (49.9261, -75.0795) projected
  line L378 (28.3222, -72.0795) -> (33.5184, -75.0795) projected
  line L379 (28.3222, -75.0795) -> (28.3222, -72.0795) projected
  arc A57 (26.3222, -75.0795) -> (28.3222, -75.0795) centre (27.3222, -75.0795) ccw projected
  line L380 (26.3222, -72.0795) -> (26.3222, -75.0795) projected
  line L381 (21.1261, -75.0795) -> (26.3222, -72.0795) projected
  line L382 (4.7184, -75.0795) -> (21.1261, -75.0795) projected
  line L383 (-0.4778, -72.0795) -> (4.7184, -75.0795) projected
  line L384 (-0.4778, -75.0795) -> (-0.4778, -72.0795) projected
  arc A58 (-2.4778, -75.0795) -> (-0.4778, -75.0795) centre (-1.4778, -75.0795) ccw projected
  line L385 (-2.4778, -72.0795) -> (-2.4778, -75.0795) projected
  line L386 (-7.6739, -75.0795) -> (-2.4778, -72.0795) projected
  line L387 (-24.0816, -75.0795) -> (-7.6739, -75.0795) projected
  line L388 (-29.2778, -72.0795) -> (-24.0816, -75.0795) projected
  line L389 (-29.2778, -75.0795) -> (-29.2778, -72.0795) projected
  arc A59 (-31.2778, -75.0795) -> (-29.2778, -75.0795) centre (-30.2778, -75.0795) ccw projected
  line L390 (-31.2778, -72.0795) -> (-31.2778, -75.0795) projected
  line L391 (-36.4739, -75.0795) -> (-31.2778, -72.0795) projected
  line L392 (-36.4739, -75.0795) -> (-44.6778, -75.0795) projected
  line L393 (-44.6778, -114.8795) -> (-44.6778, -75.0795) projected
  line L394 (-22.0739, -114.8795) -> (-44.6778, -114.8795) projected
  line L395 (-16.8778, -117.8795) -> (-22.0739, -114.8795) projected
  line L396 (-16.8778, -114.8795) -> (-16.8778, -117.8795) projected
  arc A60 (-14.8778, -114.8795) -> (-16.8778, -114.8795) centre (-15.8778, -114.8795) ccw projected
  line L397 (-14.8778, -117.8795) -> (-14.8778, -114.8795) projected
  line L398 (-9.6816, -114.8795) -> (-14.8778, -117.8795) projected
  line L399 (6.7261, -114.8795) -> (-9.6816, -114.8795) projected
  line L400 (11.9222, -117.8795) -> (6.7261, -114.8795) projected
  line L401 (11.9222, -114.8795) -> (11.9222, -117.8795) projected
  arc A61 (13.9222, -114.8795) -> (11.9222, -114.8795) centre (12.9222, -114.8795) ccw projected
  line L402 (13.9222, -117.8795) -> (13.9222, -114.8795) projected
  line L403 (19.1184, -114.8795) -> (13.9222, -117.8795) projected
  line L404 (35.5261, -114.8795) -> (19.1184, -114.8795) projected
  line L405 (40.7222, -117.8795) -> (35.5261, -114.8795) projected
  line L406 (40.7222, -114.8795) -> (40.7222, -117.8795) projected
  arc A62 (42.7222, -114.8795) -> (40.7222, -114.8795) centre (41.7222, -114.8795) ccw projected
  line L407 (42.7222, -117.8795) -> (42.7222, -114.8795) projected
  line L408 (47.9184, -114.8795) -> (42.7222, -117.8795) projected
  line L409 (64.3261, -114.8795) -> (47.9184, -114.8795) projected
  line L410 (69.5222, -117.8795) -> (64.3261, -114.8795) projected
  line L411 (69.5222, -114.8795) -> (69.5222, -117.8795) projected
  arc A63 (71.5222, -114.8795) -> (69.5222, -114.8795) centre (70.5222, -114.8795) ccw projected
  line L412 (71.5222, -117.8795) -> (71.5222, -114.8795) projected
  line L413 (76.7184, -114.8795) -> (71.5222, -117.8795) projected
  line L414 (93.1261, -114.8795) -> (76.7184, -114.8795) projected
  line L415 (98.3222, -117.8795) -> (93.1261, -114.8795) projected
  line L416 (98.3222, -114.8795) -> (98.3222, -117.8795) projected
  arc A64 (100.3222, -114.8795) -> (98.3222, -114.8795) centre (99.3222, -114.8795) ccw projected
  line L417 (100.3222, -117.8795) -> (100.3222, -114.8795) projected
  line L418 (105.5184, -114.8795) -> (100.3222, -117.8795) projected
  line L419 (121.9261, -114.8795) -> (105.5184, -114.8795) projected
  line L420 (127.1222, -117.8795) -> (121.9261, -114.8795) projected
  line L421 (127.1222, -114.8795) -> (127.1222, -117.8795) projected
  arc A65 (129.1222, -114.8795) -> (127.1222, -114.8795) centre (128.1222, -114.8795) ccw projected
  line L422 (129.1222, -117.8795) -> (129.1222, -114.8795) projected
  line L423 (134.3184, -114.8795) -> (129.1222, -117.8795) projected
  line L424 (150.7261, -114.8795) -> (134.3184, -114.8795) projected
  line L425 (155.9222, -117.8795) -> (150.7261, -114.8795) projected
  line L426 (155.9222, -114.8795) -> (155.9222, -117.8795) projected
  arc A66 (157.9222, -114.8795) -> (155.9222, -114.8795) centre (156.9222, -114.8795) ccw projected
  line L427 (157.9222, -117.8795) -> (157.9222, -114.8795) projected
  line L428 (163.1184, -114.8795) -> (157.9222, -117.8795) projected
  line L429 (179.5261, -114.8795) -> (163.1184, -114.8795) projected
  line L430 (184.7222, -117.8795) -> (179.5261, -114.8795) projected
  line L431 (184.7222, -114.8795) -> (184.7222, -117.8795) projected
  arc A67 (186.7222, -114.8795) -> (184.7222, -114.8795) centre (185.7222, -114.8795) ccw projected
  line L432 (186.7222, -117.8795) -> (186.7222, -114.8795) projected
  line L433 (191.9184, -114.8795) -> (186.7222, -117.8795) projected
  line L434 (208.3261, -114.8795) -> (191.9184, -114.8795) projected
  line L435 (213.5222, -117.8795) -> (208.3261, -114.8795) projected
  line L436 (213.5222, -114.8795) -> (213.5222, -117.8795) projected
  arc A68 (215.5222, -114.8795) -> (213.5222, -114.8795) centre (214.5222, -114.8795) ccw projected
  line L437 (215.5222, -117.8795) -> (215.5222, -114.8795) projected
  line L438 (220.7184, -114.8795) -> (215.5222, -117.8795) projected
  line L439 (237.1261, -114.8795) -> (220.7184, -114.8795) projected
  line L440 (242.3222, -117.8795) -> (237.1261, -114.8795) projected
  line L441 (242.3222, -114.8795) -> (242.3222, -117.8795) projected
  arc A69 (244.3222, -114.8795) -> (242.3222, -114.8795) centre (243.3222, -114.8795) ccw projected
  line L442 (244.3222, -117.8795) -> (244.3222, -114.8795) projected
  line L443 (249.5184, -114.8795) -> (244.3222, -117.8795) projected
  line L444 (265.9261, -114.8795) -> (249.5184, -114.8795) projected
  line L445 (271.1222, -117.8795) -> (265.9261, -114.8795) projected
  line L446 (271.1222, -114.8795) -> (271.1222, -117.8795) projected
  arc A70 (273.1222, -114.8795) -> (271.1222, -114.8795) centre (272.1222, -114.8795) ccw projected
  line L447 (273.1222, -117.8795) -> (273.1222, -114.8795) projected
  line L448 (278.3184, -114.8795) -> (273.1222, -117.8795) projected
  line L449 (294.7261, -114.8795) -> (278.3184, -114.8795) projected
  line L450 (299.9222, -117.8795) -> (294.7261, -114.8795) projected
  line L451 (299.9222, -114.8795) -> (299.9222, -117.8795) projected
  arc A71 (301.9222, -114.8795) -> (299.9222, -114.8795) centre (300.9222, -114.8795) ccw projected
  line L452 (301.9222, -117.8795) -> (301.9222, -114.8795) projected
  line L453 (307.1184, -114.8795) -> (301.9222, -117.8795) projected
  line L454 (323.5261, -114.8795) -> (307.1184, -114.8795) projected
  line L455 (328.7222, -117.8795) -> (323.5261, -114.8795) projected
  line L456 (328.7222, -114.8795) -> (328.7222, -117.8795) projected
  arc A72 (330.7222, -114.8795) -> (328.7222, -114.8795) centre (329.7222, -114.8795) ccw projected
  line L457 (330.7222, -117.8795) -> (330.7222, -114.8795) projected
  line L458 (335.9184, -114.8795) -> (330.7222, -117.8795) projected
  line L459 (352.3261, -114.8795) -> (335.9184, -114.8795) projected
  line L460 (357.5222, -117.8795) -> (352.3261, -114.8795) projected
  line L461 (357.5222, -114.8795) -> (357.5222, -117.8795) projected
  arc A73 (359.5222, -114.8795) -> (357.5222, -114.8795) centre (358.5222, -114.8795) ccw projected
  line L462 (359.5222, -117.8795) -> (359.5222, -114.8795) projected
  line L463 (364.7184, -114.8795) -> (359.5222, -117.8795) projected
  line L464 (381.1261, -114.8795) -> (364.7184, -114.8795) projected
  line L465 (386.3222, -117.8795) -> (381.1261, -114.8795) projected
  line L466 (386.3222, -114.8795) -> (386.3222, -117.8795) projected
  arc A74 (388.3222, -114.8795) -> (386.3222, -114.8795) centre (387.3222, -114.8795) ccw projected
  line L467 (388.3222, -117.8795) -> (388.3222, -114.8795) projected
  line L468 (393.5184, -114.8795) -> (388.3222, -117.8795) projected
  line L469 (409.9261, -114.8795) -> (393.5184, -114.8795) projected
  line L470 (415.1222, -117.8795) -> (409.9261, -114.8795) projected
  line L471 (415.1222, -114.8795) -> (415.1222, -117.8795) projected
  arc A75 (417.1222, -114.8795) -> (415.1222, -114.8795) centre (416.1222, -114.8795) ccw projected
  line L472 (417.1222, -117.8795) -> (417.1222, -114.8795) projected
  line L473 (422.3184, -114.8795) -> (417.1222, -117.8795) projected
  line L474 (438.7261, -114.8795) -> (422.3184, -114.8795) projected
  line L475 (443.9222, -117.8795) -> (438.7261, -114.8795) projected
  line L476 (443.9222, -114.8795) -> (443.9222, -117.8795) projected
  arc A76 (445.9222, -114.8795) -> (443.9222, -114.8795) centre (444.9222, -114.8795) ccw projected
  line L477 (445.9222, -117.8795) -> (445.9222, -114.8795) projected
  line L478 (451.1184, -114.8795) -> (445.9222, -117.8795) projected
  line L479 (467.5261, -114.8795) -> (451.1184, -114.8795) projected
  line L480 (472.7222, -117.8795) -> (467.5261, -114.8795) projected
  line L481 (472.7222, -114.8795) -> (472.7222, -117.8795) projected
  arc A77 (474.7222, -114.8795) -> (472.7222, -114.8795) centre (473.7222, -114.8795) ccw projected
  line L482 (474.7222, -117.8795) -> (474.7222, -114.8795) projected
  line L483 (479.9184, -114.8795) -> (474.7222, -117.8795) projected
  line L484 (496.3261, -114.8795) -> (479.9184, -114.8795) projected
  line L485 (501.5222, -117.8795) -> (496.3261, -114.8795) projected
  line L486 (501.5222, -114.8795) -> (501.5222, -117.8795) projected
  arc A78 (503.5222, -114.8795) -> (501.5222, -114.8795) centre (502.5222, -114.8795) ccw projected
  line L487 (503.5222, -117.8795) -> (503.5222, -114.8795) projected
  line L488 (508.7184, -114.8795) -> (503.5222, -117.8795) projected
  line L489 (525.1261, -114.8795) -> (508.7184, -114.8795) projected
  line L490 (530.3222, -117.8795) -> (525.1261, -114.8795) projected
  line L491 (530.3222, -114.8795) -> (530.3222, -117.8795) projected
  arc A79 (532.3222, -114.8795) -> (530.3222, -114.8795) centre (531.3222, -114.8795) ccw projected
  line L492 (-15.2778, -103.9795) -> (-9.2778, -103.9795) projected
  line L493 (-9.2778, -103.9795) -> (-9.2778, -109.9795) projected
  line L494 (-9.2778, -109.9795) -> (-15.2778, -109.9795) projected
  line L495 (-15.2778, -109.9795) -> (-15.2778, -103.9795) projected
  line L496 (-15.2778, -85.9795) -> (-15.2778, -79.9795) projected
  line L497 (-15.2778, -79.9795) -> (-9.2778, -79.9795) projected
  line L498 (-9.2778, -79.9795) -> (-9.2778, -85.9795) projected
  line L499 (-9.2778, -85.9795) -> (-15.2778, -85.9795) projected
  line L500 (42.3222, -103.9795) -> (48.3222, -103.9795) projected
  line L501 (48.3222, -103.9795) -> (48.3222, -109.9795) projected
  line L502 (48.3222, -109.9795) -> (42.3222, -109.9795) projected
  line L503 (42.3222, -109.9795) -> (42.3222, -103.9795) projected
  line L504 (42.3222, -85.9795) -> (42.3222, -79.9795) projected
  line L505 (42.3222, -79.9795) -> (48.3222, -79.9795) projected
  line L506 (48.3222, -79.9795) -> (48.3222, -85.9795) projected
  line L507 (48.3222, -85.9795) -> (42.3222, -85.9795) projected
  line L508 (99.9222, -103.9795) -> (105.9222, -103.9795) projected
  line L509 (105.9222, -103.9795) -> (105.9222, -109.9795) projected
  line L510 (105.9222, -109.9795) -> (99.9222, -109.9795) projected
  line L511 (99.9222, -109.9795) -> (99.9222, -103.9795) projected
  line L512 (99.9222, -85.9795) -> (99.9222, -79.9795) projected
  line L513 (99.9222, -79.9795) -> (105.9222, -79.9795) projected
  line L514 (105.9222, -79.9795) -> (105.9222, -85.9795) projected
  line L515 (105.9222, -85.9795) -> (99.9222, -85.9795) projected
  line L516 (157.5222, -103.9795) -> (163.5222, -103.9795) projected
  line L517 (163.5222, -103.9795) -> (163.5222, -109.9795) projected
  line L518 (163.5222, -109.9795) -> (157.5222, -109.9795) projected
  line L519 (157.5222, -109.9795) -> (157.5222, -103.9795) projected
  line L520 (157.5222, -85.9795) -> (157.5222, -79.9795) projected
  line L521 (157.5222, -79.9795) -> (163.5222, -79.9795) projected
  line L522 (163.5222, -79.9795) -> (163.5222, -85.9795) projected
  line L523 (163.5222, -85.9795) -> (157.5222, -85.9795) projected
  line L524 (215.1222, -103.9795) -> (221.1222, -103.9795) projected
  line L525 (221.1222, -103.9795) -> (221.1222, -109.9795) projected
  line L526 (221.1222, -109.9795) -> (215.1222, -109.9795) projected
  line L527 (215.1222, -109.9795) -> (215.1222, -103.9795) projected
  line L528 (215.1222, -85.9795) -> (215.1222, -79.9795) projected
  line L529 (215.1222, -79.9795) -> (221.1222, -79.9795) projected
  line L530 (221.1222, -79.9795) -> (221.1222, -85.9795) projected
  line L531 (221.1222, -85.9795) -> (215.1222, -85.9795) projected
  line L532 (272.7222, -103.9795) -> (278.7222, -103.9795) projected
  line L533 (278.7222, -103.9795) -> (278.7222, -109.9795) projected
  line L534 (278.7222, -109.9795) -> (272.7222, -109.9795) projected
  line L535 (272.7222, -109.9795) -> (272.7222, -103.9795) projected
  line L536 (272.7222, -85.9795) -> (272.7222, -79.9795) projected
  line L537 (272.7222, -79.9795) -> (278.7222, -79.9795) projected
  line L538 (278.7222, -79.9795) -> (278.7222, -85.9795) projected
  line L539 (278.7222, -85.9795) -> (272.7222, -85.9795) projected
  line L540 (330.3222, -103.9795) -> (336.3222, -103.9795) projected
  line L541 (336.3222, -103.9795) -> (336.3222, -109.9795) projected
  line L542 (336.3222, -109.9795) -> (330.3222, -109.9795) projected
  line L543 (330.3222, -109.9795) -> (330.3222, -103.9795) projected
  line L544 (330.3222, -85.9795) -> (330.3222, -79.9795) projected
  line L545 (330.3222, -79.9795) -> (336.3222, -79.9795) projected
  line L546 (336.3222, -79.9795) -> (336.3222, -85.9795) projected
  line L547 (336.3222, -85.9795) -> (330.3222, -85.9795) projected
  line L548 (387.9222, -103.9795) -> (393.9222, -103.9795) projected
  line L549 (393.9222, -103.9795) -> (393.9222, -109.9795) projected
  line L550 (393.9222, -109.9795) -> (387.9222, -109.9795) projected
  line L551 (387.9222, -109.9795) -> (387.9222, -103.9795) projected
  line L552 (387.9222, -85.9795) -> (387.9222, -79.9795) projected
  line L553 (387.9222, -79.9795) -> (393.9222, -79.9795) projected
  line L554 (393.9222, -79.9795) -> (393.9222, -85.9795) projected
  line L555 (393.9222, -85.9795) -> (387.9222, -85.9795) projected
  line L556 (445.5222, -103.9795) -> (451.5222, -103.9795) projected
  line L557 (451.5222, -103.9795) -> (451.5222, -109.9795) projected
  line L558 (451.5222, -109.9795) -> (445.5222, -109.9795) projected
  line L559 (445.5222, -109.9795) -> (445.5222, -103.9795) projected
  line L560 (445.5222, -85.9795) -> (445.5222, -79.9795) projected
  line L561 (445.5222, -79.9795) -> (451.5222, -79.9795) projected
  line L562 (451.5222, -79.9795) -> (451.5222, -85.9795) projected
  line L563 (451.5222, -85.9795) -> (445.5222, -85.9795) projected
  line L564 (503.1222, -103.9795) -> (509.1222, -103.9795) projected
  line L565 (509.1222, -103.9795) -> (509.1222, -109.9795) projected
  line L566 (509.1222, -109.9795) -> (503.1222, -109.9795) projected
  line L567 (503.1222, -109.9795) -> (503.1222, -103.9795) projected
  line L568 (503.1222, -85.9795) -> (503.1222, -79.9795) projected
  line L569 (503.1222, -79.9795) -> (509.1222, -79.9795) projected
  line L570 (509.1222, -79.9795) -> (509.1222, -85.9795) projected
  line L571 (509.1222, -85.9795) -> (503.1222, -85.9795) projected
  point P0 (0, 0)
extrude "Extrusion1" add sketch "Sketch1" along normal blind 6 and the other way blind 6 contours L206 L207 L208 L209 | L496 L497 L498 L499
sketch "Sketch2" plane through (-15.2778, -79.9795, 6) normal (0, 1, 0) x (1, 0, 0)
  line L0 (6, 0) -> (0, 0) projected
  line L1 (6, 12) -> (6, 0) projected
  line L2 (0, 0) -> (6, 0)
  line L3 (6, 0) -> (6, 6)
  line L4 (6, 6) -> (0, 6)
  line L5 (0, 6) -> (0, 0)
  point P0 (15.2778, 6)
  dimension "d4" = 6
  constraints: 8 end point, 2 parallel, 1 horizontal, 1 midpoint, 1 perpendicular
  measures "d4" distance of L4.end L3.end
extrude "Extrusion2" add sketch "Sketch2" along normal up to next
body "Solid1"
